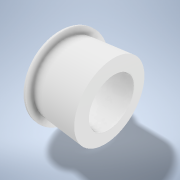
# Autodesk Inventor part: Rolle_schieber
Saved by Autodesk Inventor 2021 (Build 250183000, 183)
## iProperties
Created: 2022-06-26
Part Number: Rolle_schieber
Material: PC/ABS-Kunststoff
Document SubType Name: Modeling
Designer: adria
Mass: 4.08443 g
Surface Area: 54.6637 cm^2
Volume: 11.4323 cm^3
Density: 0.357273 g/cm^3
Appearance: Glatt - Weiß
Author: adria
Autodesk Inventor part; units mm, degrees
ref_plane "YZ Plane" through (0, 0, 0) normal (1, 0, 0) x (0, 1, 0)
ref_plane "XZ Plane" through (0, 0, 0) normal (0, 1, 0) x (-1, 0, 0)
ref_plane "XY Plane" through (0, 0, 0) normal (0, 0, 1) x (1, 0, 0)
sketch "Skizze1" plane through (0, 0, 0) normal (1, 0, 0) x (0, 1, 0)
  circle A0 centre (0, 0) radius 20
  dimension "d0" = 40
  constraints: 1 centre point, 1 coincident
  measures "d0" diameter of A0
extrude "Extrusion1" add sketch "Skizze1" along normal blind 1
sketch "Skizze2" plane through (1, 0, 0) normal (1, 0, 0) x (0, 0, -1)
  circle A0 centre (0, 0) radius 20 projected
  circle A1 centre (0, 0) radius 17
  dimension "d3" = 34
  constraints: 1 centre point, 1 coincident
  measures "d3" diameter of A1
extrude "Extrusion2" add sketch "Skizze2" along normal blind 20 contours A1
sketch "Skizze5" plane through (0, 0, 0) normal (-1, 0, 0) x (0, 0, 1)
  circle A0 centre (0, 0) radius 20 projected
  circle A1 centre (0, 0) radius 5
  dimension "d12" = 10
  constraints: 1 centre point, 1 coincident
  measures "d12" diameter of A1
extrude "Extrusion5" add sketch "Skizze5" along normal blind 10 contours A1
sketch "Skizze6" plane through (21, 0, 0) normal (1, 0, 0) x (0, 0, -1)
  circle A0 centre (0, 0) radius 17 projected
  circle A1 centre (0, 0) radius 11
  dimension "d15" = 22
  constraints: 1 centre point, 1 coincident
  measures "d15" diameter of A1
extrude "Extrusion6" cut sketch "Skizze6" against normal through all contours A1
